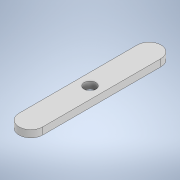
# Autodesk Inventor part: locker
Saved by Autodesk Inventor 2021 (Build 250183000, 183)
## iProperties
Created: 2020-06-13
Part Number: locker
Material: Generic
Document SubType Name: Modeling
Designer: Yatekii
Density: 1 g/cm^3
Appearance: Default
Author: Yatekii
Autodesk Inventor part; units mm, degrees
ref_plane "YZ Plane" through (0, 0, 0) normal (1, 0, 0) x (0, 1, 0)
ref_plane "XZ Plane" through (0, 0, 0) normal (0, 1, 0) x (-1, 0, 0)
ref_plane "XY Plane" through (0, 0, 0) normal (0, 0, 1) x (1, 0, 0)
sketch "Sketch1" plane through (0, 0, 0) normal (0, 1, 0) x (-1, 0, 0)
  circle A0 centre (0, 0) radius 2.5085
  line L0 (0, -25) -> (0, 25) construction
  line L1 (5, -25) -> (5, 25)
  line L2 (-5, 25) -> (-5, -25)
  arc A1 (-5, -25) -> (5, -25) centre (0, -25) ccw
  arc A2 (5, 25) -> (-5, 25) centre (0, 25) ccw
  dimension "d0" = 5.017
  dimension "d1" = 25
  dimension "d2" = 10
  constraints: 8 end point, 4 point on circle, 4 tangent, 3 centre point, 1 coincident, 1 midpoint, 1 parallel, 1 vertical
  measures "d0" diameter of A0
  measures "d1" distance of A0.centre L0.end
  measures "d2" diameter of A2
extrude "Extrusion1" add sketch "Sketch1" along normal blind 3
body "Solid1"
